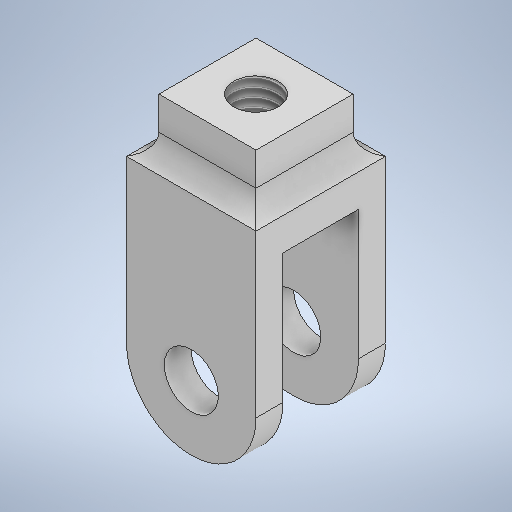
# Autodesk Inventor part: 2063
Saved by Autodesk Inventor 2025 (Build 290162010, 162A)
## iProperties
Created: 2024-05-30
Part Number: 2063
Material: Generic
Document SubType Name: Modeling
Designer: Fabri
Density: 1 g/cm^3
Appearance: Default
Author: Fabri
Autodesk Inventor part; units mm, degrees
note: some values were not read from the file. Chosen so that the rebuilt part matches the saved one: direction of "Hole1"; direction of "Hole2".
ref_plane "YZ Plane" through (0, 0, 0) normal (1, 0, 0) x (0, 1, 0)
ref_plane "XZ Plane" through (0, 0, 0) normal (0, 1, 0) x (-1, 0, 0)
ref_plane "XY Plane" through (0, 0, 0) normal (0, 0, 1) x (1, 0, 0)
sketch "Sketch1" plane through (0, 0, 0) normal (0, 1, 0) x (-1, 0, 0)
  line L0 (0, 0) -> (12, 0)
  line L1 (12, 0) -> (12, -15)
  line L2 (12, -15) -> (0, -15)
  line L3 (0, -15) -> (0, 0)
  dimension "d0" = 12
  dimension "d1" = 15
  constraints: 8 end point, 2 parallel, 1 horizontal, 1 perpendicular
  measures "d0" distance between parallel lines of L3 L1
  measures "d1" distance between parallel lines of L0 L2
extrude "Extrusion1" add sketch "Sketch1" along normal blind 12
sketch "Sketch4" plane through (0, 0, 0) normal (0, -1, 0) x (1, 0, 0)
  line L0 (0, -15) -> (-12, -15) projected
  arc A0 (-12, -15) -> (0, -15) centre (-6, -15) ccw
  point P0 (0, 0)
  point P1 (-6, -15)
  constraints: 2 point on circle, 1 centre point, 1 coincident, 1 midpoint
extrude "Extrusion2" add sketch "Sketch4" against normal up to surface (12 mm away)
sketch "Sketch5" plane through (0, 0, 0) normal (1, 0, 0) x (0, 0, -1)
  line L0 (3, 9.5) -> (21, 9.5)
  line L1 (21, 9.5) -> (21, 2.5)
  line L2 (21, 2.5) -> (3, 2.5)
  line L3 (3, 2.5) -> (3, 9.5)
  line L4 (15, 12) -> (15, 12) projected
  line L5 (15, 0) -> (15, 12) projected
  line L6 (15, 0) -> (15, 0) projected
  line L7 (15, 0) -> (15, 12) projected
  line L8 (21, 0) -> (21, 12) projected
  line L9 (0, 0) -> (0, 12) projected
  point P0 (21, 6)
  point P1 (3, 6)
  point P2 (0, 6)
  dimension "d8" = 18
  dimension "d9" = 7
  constraints: 8 end point, 4 midpoint, 2 parallel, 1 horizontal, 1 horizontal alignment, 1 perpendicular
  measures "d8" distance between parallel lines of L1 L3
  measures "d9" distance between parallel lines of L2 L0
extrude "Extrusion3" cut sketch "Sketch5" against normal up to surface (12 mm away)
sketch "Sketch6" plane through (0, 12, 0) normal (0, 1, 0) x (1, 0, 0)
  arc A0 (0, 15) -> (-12, 15) centre (-6, 15) ccw projected
  point P0 (0, 0)
  constraints: 1 coincident
hole "Hole1" at (-6, 12, -15) direction (0, -1, 0) diameter 5 depth 12
sketch "Sketch7" plane through (-12, 0, 0) normal (0, 0, 1) x (1, 0, 0)
  line L0 (10.5, 1.5) -> (1.5, 1.5)
  line L1 (1.5, 1.5) -> (1.5, 10.5)
  line L2 (1.5, 10.5) -> (10.5, 10.5)
  line L3 (10.5, 10.5) -> (10.5, 1.5)
  line L4 (0, 0) -> (0, 12) projected
  line L5 (0, 0) -> (12, 0) projected
  point P0 (1.5, 6)
  point P1 (0, 6)
  point P2 (6, 1.5)
  point P3 (6, 0)
  dimension "d19" = 9
  dimension "d20" = 9
  constraints: 8 end point, 4 midpoint, 2 parallel, 1 horizontal, 1 horizontal alignment, 1 perpendicular, 1 vertical alignment
  measures "d19" distance between parallel lines of L1 L3
  measures "d20" distance between parallel lines of L2 L0
extrude "Extrusion4" add sketch "Sketch7" along normal blind 5
fillet "Fillet1" radius 2 4 edges at (-6, 1.5, 0) (-10.5, 6, 0) (-6, 10.5, 0) (-1.5, 6, 0)
sketch "Sketch8" plane through (-12, 0, 5) normal (0, 0, 1) x (1, 0, 0)
  line L0 (10.5, 1.5) -> (10.5, 10.5) projected
  line L1 (1.5, 1.5) -> (10.5, 1.5) projected
  point P0 (12, 0)
  point P1 (6, 6)
  point P2 (10.5, 6)
  point P3 (6, 1.5)
  constraints: 2 midpoint, 1 horizontal alignment, 1 vertical alignment
hole "Hole2" at (-6, 6, 5) direction (0, 0, -1) diameter 4.134 depth 8 thread size "M5x0.8" class "6H" standard "ISO Metric profile"
body "Solid1"
